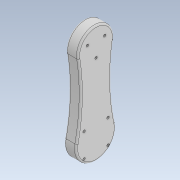
# Autodesk Inventor part: leg_demo_8
Saved by Autodesk Inventor 2020 (Build 240168000, 168)
## iProperties
Created: 2020-12-17
Part Number: leg_demo_8
Material: Generic
Document SubType Name: Modeling
Designer: DELL
Density: 1 g/cm^3
Appearance: Default
Author: DELL
Autodesk Inventor part; units mm, degrees
ref_plane "YZ Plane" through (0, 0, 0) normal (1, 0, 0) x (0, 1, 0)
ref_plane "XZ Plane" through (0, 0, 0) normal (0, 1, 0) x (-1, 0, 0)
ref_plane "XY Plane" through (0, 0, 0) normal (0, 0, 1) x (1, 0, 0)
sketch "Sketch1" plane through (0, 0, 0) normal (1, 0, 0) x (0, 1, 0)
  circle A0 centre (0, 0) radius 12.5 construction
  line L0 (6.25, 10.8253) -> (0, 0) construction
  line L1 (0, 0) -> (-12.5, 0) construction
  line L2 (0, 0) -> (6.25, -10.8253) construction
  line L3 (0, 12.5) -> (0, -12.5) construction
  circle A1 centre (6.25, 10.8253) radius 1.5
  circle A2 centre (6.25, -10.8253) radius 1.5
  circle A3 centre (-12.5, 0) radius 1.5
  circle A4 centre (0, 0) radius 22.5
  circle A5 centre (-100, 0) radius 25
  circle A6 centre (-100, 0) radius 21.2132 construction
  arc A7 (-94.8324, 24.4601) -> (-3.5634, 22.216) centre (-43.1562, 269.0609) ccw
  arc A8 (-3.5634, -22.216) -> (-94.8324, -24.4601) centre (-43.1562, -269.0609) ccw
  line L4 (-100, 25) -> (-100, -25) construction
  line L5 (-75, 0) -> (-125, 0) construction
  line L6 (-82.3223, 17.6777) -> (-117.6777, -17.6777) construction
  line L7 (-82.3223, -17.6777) -> (-117.6777, 17.6777) construction
  circle A9 centre (-85, 15) radius 1.5
  circle A10 centre (-85, -15) radius 1.5
  circle A11 centre (-115, -15) radius 1.5
  circle A12 centre (-115, 15) radius 1.5
  point P0 (-94.8324, -24.4601)
  point P1 (-3.5634, -22.216)
  dimension "d4" = 45
  dimension "d6" = 50
  dimension "d0" = 25
  dimension "d1" = 30
  dimension "d2" = 30
  dimension "d3" = 3
  dimension "d8" = 100
  dimension "d9" = 500
  dimension "d10" = 45
  dimension "d11" = 45
  dimension "d12" = 3
  dimension "d15" = 30
  constraints: 16 end point, 13 point on circle, 11 centre point, 9 midpoint, 6 coincident, 5 equal radius, 4 point on line, 3 symmetric about line, 2 vertical, 1 horizontal, 1 horizontal alignment, 1 perpendicular, 17 other
  measures "d0" diameter of A0
  measures "d1" angle of L3 L0
  measures "d2" angle of L3 L2
  measures "d3" diameter of A1
  measures "d8" distance of point (-100, 0) point (0, 0)
  measures "d9" diameter of A7
  measures "d10" angle of L4 L6
  measures "d11" angle of L4 L7
  measures "d12" diameter of A9
  measures "d15" distance of A12.centre A9.centre
extrude "Extrusion1" add sketch "Sketch1" along normal blind 15
fillet "Fillet1" radius 2 8 edges at (15, -49.3012, 19.1365) (15, -125, 0) (15, -49.3012, -19.1365) (15, 22.5, 0) (0, -49.3012, 19.1365) (0, -125, 0) (0, -49.3012, -19.1365) (0, 22.5, 0)
body "Solid1"
